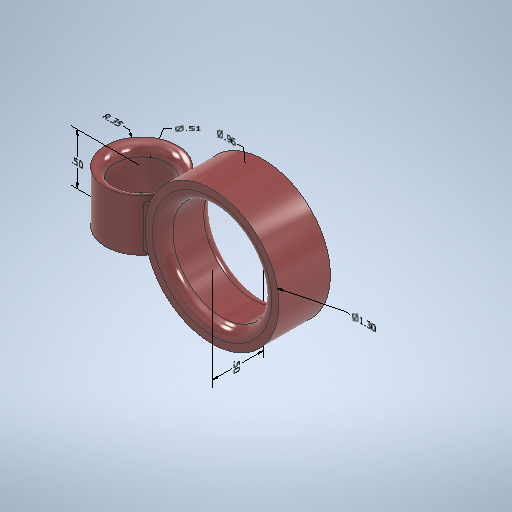
# Autodesk Inventor part: motor-dowel
Saved by Autodesk Inventor 2025.2 (Build 292293000, 293)
## iProperties
Created: 2025-04-17
Part Number: motor-dowel
Material: Generic
Document SubType Name: Modeling
Designer: 3lin2
Density: 1 g/cm^3
Appearance: Default
Author: 3lin2
Autodesk Inventor part; units mm, degrees
ref_plane "YZ Plane" through (0, 0, 0) normal (1, 0, 0) x (0, 1, 0)
ref_plane "XZ Plane" through (0, 0, 0) normal (0, 1, 0) x (-1, 0, 0)
sketch "Sketch1" plane through (0, 0, 0) normal (0, 1, 0) x (-1, 0, 0)
  circle A0 centre (0, 0) radius 6.477
  circle A1 centre (0, 0) radius 8.89
  dimension "d0" = 12.954
  dimension "d1" = 17.78
  constraints: 2 centre point, 2 coincident
  measures "d0" diameter of A0
  measures "d1" diameter of A1
extrude "Extrusion1" add sketch "Sketch1" along normal blind 12.7
ref_plane "Work Plane1" through (0, 6.35, 0) normal (0, -1, 0) x (1, 0, 0)
sketch "Sketch2" plane through (0, 6.35, 0) normal (0, -1, 0) x (1, 0, 0)
  line L0 (8.89, 12.7) -> (8.89, -12.7)
  circle A0 centre (0, 0) radius 8.89 projected
  line L1 (0, 0) -> (12.7, 0)
  dimension "d4" = 25.4
  dimension "d5" = 8.89
  dimension "d6" = 12.7
  dimension "d7" = 12.7
  constraints: 4 end point, 1 horizontal, 1 vertical
  measures "d4" distance of L0.start L0.end
  measures "d5" distance from line of L1.start L0
  measures "d6" vertical distance of L0.end point (0, 0)
  measures "d7" distance of L1.start L1.end
ref_plane "Work Plane3" through (0, 6.35, 0) normal (0, 0, -1) x (1, 0, 0)
sketch "Sketch5" plane through (0, 6.35, 0) normal (0, 0, -1) x (1, 0, 0)
  line L0 (-8.89, -6.35) -> (8.89, -6.35) projected
  circle A0 centre (23.7435, 0) radius 12.192
  circle A1 centre (23.7435, 0) radius 16.51
  point P0 (0, 6.35)
  dimension "d10" = 24.384
  dimension "d11" = 6.35
  dimension "d12" = 33.02
  constraints: 2 centre point, 1 coincident
  measures "d10" diameter of A0
  measures "d11" distance from line of L0 A0.centre
  measures "d12" diameter of A1
extrude "Extrusion2" add sketch "Sketch5" along normal mid plane 12.7
fillet "Fillet1" radius 2.54 4 edges at (11.5515, 6.35, 6.35) (11.5515, 6.35, -6.35) (6.477, 0, 0) (6.477, 12.7, 0)
sketch "Sketch6" plane through (0, 6.35, 0) normal (0, -1, 0) x (1, 0, 0)
  line L0 (7.2335, -6.35) -> (40.2535, -6.35) projected
  line L1 (9.042, -6.35) -> (6.8677, -6.35)
  line L2 (6.8677, -6.35) -> (6.8677, 6.3466)
  line L3 (6.8677, 6.3466) -> (9.042, 6.3466)
  line L4 (9.042, 6.3466) -> (9.042, -6.35)
  point P0 (0, 0)
  constraints: 8 end point, 2 parallel, 1 horizontal, 1 perpendicular, 1 point on line
extrude "Extrusion3" add sketch "Sketch6" along normal mid plane 10.16
body "Solid1"
